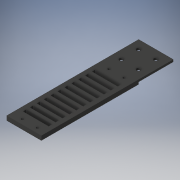
# Autodesk Inventor part: Base Right Front Panel
Saved by Autodesk Inventor 2019 (Build 230136000, 136)
## iProperties
Created: 2018-12-04
Part Number: Base Right Front Panel
Material: Generic
Document SubType Name: Modeling
Designer: Keith
Density: 1 g/cm^3
Appearance: Default
Author: Keith
## iProperties of the stored document Base Right Front Panel_3DPrint.ipt
Created: 2018-12-04
Part Number: Base Right Front Panel_3DPrint
Material: Generic
Document SubType Name: Modeling
Designer: Keith
Density: 1 g/cm^3
Appearance: Default
Author: Keith
Autodesk Inventor part; units mm, degrees
ref_plane "YZ Plane" through (0, 0, 0) normal (1, 0, 0) x (0, 1, 0)
ref_plane "XZ Plane" through (0, 0, 0) normal (0, 1, 0) x (-1, 0, 0)
ref_plane "XY Plane" through (0, 0, 0) normal (0, 0, 1) x (1, 0, 0)
sketch "Sketch1" plane through (0, 0, 0) normal (0, 1, 0) x (-1, 0, 0)
  line L0 (0, 0) -> (40, 0)
  line L1 (40, 0) -> (40, -152.8)
  line L2 (40, -152.8) -> (0, -152.8)
  line L3 (0, -152.8) -> (0, 0)
  circle A0 centre (30, -122.8) radius 2.5
  circle A1 centre (30, -142.8) radius 2.5
  circle A2 centre (10, -122.8) radius 2.5
  circle A3 centre (10, -142.8) radius 2.5
  line L4 (5, -97.55) -> (35, -97.55)
  line L5 (35, -97.55) -> (35, -93.55)
  line L6 (35, -93.55) -> (5, -93.55)
  line L7 (5, -93.55) -> (5, -97.55)
  line L8 (5, -89.55) -> (35, -89.55)
  line L9 (35, -89.55) -> (35, -85.55)
  line L10 (35, -85.55) -> (5, -85.55)
  line L11 (5, -85.55) -> (5, -89.55)
  line L12 (5, -81.55) -> (35, -81.55)
  line L13 (35, -81.55) -> (35, -77.55)
  line L14 (35, -77.55) -> (5, -77.55)
  line L15 (5, -77.55) -> (5, -81.55)
  line L16 (5, -73.55) -> (35, -73.55)
  line L17 (35, -73.55) -> (35, -69.55)
  line L18 (35, -69.55) -> (5, -69.55)
  line L19 (5, -69.55) -> (5, -73.55)
  line L20 (5, -65.55) -> (35, -65.55)
  line L21 (35, -65.55) -> (35, -61.55)
  line L22 (35, -61.55) -> (5, -61.55)
  line L23 (5, -61.55) -> (5, -65.55)
  line L24 (5, -57.55) -> (35, -57.55)
  line L25 (35, -57.55) -> (35, -53.55)
  line L26 (35, -53.55) -> (5, -53.55)
  line L27 (5, -53.55) -> (5, -57.55)
  line L28 (5, -49.55) -> (35, -49.55)
  line L29 (35, -49.55) -> (35, -45.55)
  line L30 (35, -45.55) -> (5, -45.55)
  line L31 (5, -45.55) -> (5, -49.55)
  line L32 (5, -41.55) -> (35, -41.55)
  line L33 (35, -41.55) -> (35, -37.55)
  line L34 (35, -37.55) -> (5, -37.55)
  line L35 (5, -37.55) -> (5, -41.55)
  line L36 (5, -33.55) -> (35, -33.55)
  line L37 (35, -33.55) -> (35, -29.55)
  line L38 (35, -29.55) -> (5, -29.55)
  line L39 (5, -29.55) -> (5, -33.55)
  line L40 (5, -25.55) -> (35, -25.55)
  line L41 (35, -25.55) -> (35, -21.55)
  line L42 (35, -21.55) -> (5, -21.55)
  line L43 (5, -21.55) -> (5, -25.55)
  line L44 (5, -17.55) -> (35, -17.55)
  line L45 (35, -17.55) -> (35, -13.55)
  line L46 (35, -13.55) -> (5, -13.55)
  line L47 (5, -13.55) -> (5, -17.55)
  dimension "d0" = 40
  dimension "d1" = 152.8
  dimension "d2" = 5
  dimension "d3" = 5
  dimension "d4" = 5
  dimension "d5" = 5
  dimension "d6" = 10
  dimension "d7" = 0
  dimension "d8" = 20
  dimension "d11" = 30
  dimension "d12" = 20
  dimension "d13" = 30
  dimension "d14" = 10
  dimension "d15" = 0
  dimension "d16" = 30
  dimension "d18" = 55.25
  dimension "d31" = 30
  dimension "d33" = 30
  dimension "d35" = 30
  dimension "d37" = 30
  dimension "d39" = 30
  dimension "d41" = 30
  dimension "d43" = 30
  dimension "d45" = 30
  dimension "d47" = 30
  dimension "d49" = 30
  constraints: 96 end point, 24 parallel, 12 horizontal, 12 perpendicular, 4 centre point
  measures "d0" distance of L1.end L2.end
  measures "d1" distance of L0.end L1.end
  measures "d2" diameter of A0
  measures "d3" diameter of A1
  measures "d4" diameter of A2
  measures "d5" diameter of A3
  measures "d6" distance from line of L1 A0.centre
  measures "d7" horizontal distance of A0.centre A1.centre
  measures "d8" distance of A0.centre A2.centre
  measures "d11" distance from line of L2 A0.centre
  measures "d12" distance of A1.centre A0.centre
  measures "d13" distance from line of L2 A2.centre
  measures "d14" distance from line of L2 A3.centre
  measures "d15" horizontal distance of A2.centre A3.centre
  measures "d16" distance of L6.end L5.end
  measures "d18" distance between parallel lines of L2 L4
  measures "d31" distance of L10.end L9.end
  measures "d33" distance of L14.end L13.end
  measures "d35" distance of L18.end L17.end
  measures "d37" distance of L22.end L21.end
  measures "d39" distance of L27.start L25.end
  measures "d41" distance of L31.start L29.end
  measures "d43" distance of L35.start L33.end
  measures "d45" distance of L39.start L37.end
  measures "d47" distance of L43.start L41.end
  measures "d49" distance of L47.start L45.end
extrude "Extrusion1" add sketch "Sketch1" along normal blind 5
sketch "Sketch2" plane through (0, 5, 0) normal (0, 1, 0) x (1, 0, 0)
  line L0 (-5, 17.55) -> (-5, 13.55) projected
  line L1 (-5, 13.55) -> (-35, 13.55) projected
  line L2 (-35, 13.55) -> (-35, 17.55) projected
  line L3 (-35, 17.55) -> (-5, 17.55) projected
  line L4 (-5, 25.55) -> (-5, 21.55) projected
  line L5 (-5, 21.55) -> (-35, 21.55) projected
  line L6 (-35, 21.55) -> (-35, 25.55) projected
  line L7 (-35, 25.55) -> (-5, 25.55) projected
  line L8 (-5, 33.55) -> (-5, 29.55) projected
  line L9 (-5, 29.55) -> (-35, 29.55) projected
  line L10 (-35, 29.55) -> (-35, 33.55) projected
  line L11 (-35, 33.55) -> (-5, 33.55) projected
  line L12 (-5, 41.55) -> (-5, 37.55) projected
  line L13 (-5, 37.55) -> (-35, 37.55) projected
  line L14 (-35, 37.55) -> (-35, 41.55) projected
  line L15 (-35, 41.55) -> (-5, 41.55) projected
  line L16 (-5, 49.55) -> (-5, 45.55) projected
  line L17 (-5, 45.55) -> (-35, 45.55) projected
  line L18 (-35, 45.55) -> (-35, 49.55) projected
  line L19 (-35, 49.55) -> (-5, 49.55) projected
  line L20 (-5, 57.55) -> (-5, 53.55) projected
  line L21 (-5, 53.55) -> (-35, 53.55) projected
  line L22 (-35, 53.55) -> (-35, 57.55) projected
  line L23 (-35, 57.55) -> (-5, 57.55) projected
  line L24 (-5, 65.55) -> (-5, 61.55) projected
  line L25 (-5, 61.55) -> (-35, 61.55) projected
  line L26 (-35, 61.55) -> (-35, 65.55) projected
  line L27 (-35, 65.55) -> (-5, 65.55) projected
  line L28 (-5, 73.55) -> (-5, 69.55) projected
  line L29 (-5, 69.55) -> (-35, 69.55) projected
  line L30 (-35, 69.55) -> (-35, 73.55) projected
  line L31 (-35, 73.55) -> (-5, 73.55) projected
  line L32 (-5, 81.55) -> (-5, 77.55) projected
  line L33 (-5, 77.55) -> (-35, 77.55) projected
  line L34 (-35, 77.55) -> (-35, 81.55) projected
  line L35 (-35, 81.55) -> (-5, 81.55) projected
  line L36 (-5, 89.55) -> (-5, 85.55) projected
  line L37 (-5, 85.55) -> (-35, 85.55) projected
  line L38 (-35, 85.55) -> (-35, 89.55) projected
  line L39 (-35, 89.55) -> (-5, 89.55) projected
  line L40 (-5, 97.55) -> (-5, 93.55) projected
  line L41 (-5, 93.55) -> (-35, 93.55) projected
  line L42 (-35, 93.55) -> (-35, 97.55) projected
  line L43 (-35, 97.55) -> (-5, 97.55) projected
  circle A0 centre (-10, 142.8) radius 2.5 projected
  circle A1 centre (-10, 122.8) radius 2.5 projected
  circle A2 centre (-30, 142.8) radius 2.5 projected
  circle A3 centre (-30, 122.8) radius 2.5 projected
  line L44 (-40, 0) -> (0, 0) projected
  line L45 (0, 0) -> (0, 152.8) projected
  line L46 (0, 152.8) -> (-40, 152.8) projected
  line L47 (-40, 152.8) -> (-40, 0) projected
  circle A4 centre (-27.5, 5.625) radius 1.5
  circle A5 centre (-10, 5.625) radius 1.5
  circle A6 centre (-27.5, 105.925) radius 1.5
  circle A7 centre (-10, 105.925) radius 1.5
  dimension "d53" = 3
  dimension "d54" = 3
  dimension "d55" = 3
  dimension "d56" = 3
  dimension "d57" = 12.5
  dimension "d58" = 10
  dimension "d59" = 12.5
  dimension "d60" = 10
  dimension "d61" = 5.625
  dimension "d62" = 5.625
  dimension "d63" = 46.875
  dimension "d64" = 46.875
  constraints: 4 centre point
  measures "d53" diameter of A4
  measures "d54" diameter of A5
  measures "d55" diameter of A6
  measures "d56" diameter of A7
  measures "d57" distance from line of L47 A4.centre
  measures "d58" distance from line of L45 A5.centre
  measures "d59" distance from line of L47 A6.centre
  measures "d60" distance from line of L45 A7.centre
  measures "d61" distance from line of L44 A4.centre
  measures "d62" distance from line of L44 A5.centre
  measures "d63" distance from line of L46 A6.centre
  measures "d64" distance from line of L46 A7.centre
extrude "Extrusion2" cut sketch "Sketch2" against normal blind 5 contours A4 | A5 | A6 | A7
sketch "Sketch3" plane through (0, 0, 0) normal (0, -1, 0) x (1, 0, 0)
  circle A0 centre (-27.5, -105.925) radius 1.5 projected
  circle A1 centre (-27.5, -5.625) radius 1.5 projected
  circle A2 centre (-10, -5.625) radius 1.5 projected
  circle A3 centre (-10, -105.925) radius 1.5 projected
  line L0 (-5, -13.55) -> (-5, -17.55) projected
  line L1 (-5, -17.55) -> (-35, -17.55) projected
  line L2 (-35, -17.55) -> (-35, -13.55) projected
  line L3 (-35, -13.55) -> (-5, -13.55) projected
  line L4 (-5, -21.55) -> (-5, -25.55) projected
  line L5 (-5, -25.55) -> (-35, -25.55) projected
  line L6 (-35, -25.55) -> (-35, -21.55) projected
  line L7 (-35, -21.55) -> (-5, -21.55) projected
  line L8 (-5, -29.55) -> (-5, -33.55) projected
  line L9 (-5, -33.55) -> (-35, -33.55) projected
  line L10 (-35, -33.55) -> (-35, -29.55) projected
  line L11 (-35, -29.55) -> (-5, -29.55) projected
  line L12 (-5, -37.55) -> (-5, -41.55) projected
  line L13 (-5, -41.55) -> (-35, -41.55) projected
  line L14 (-35, -41.55) -> (-35, -37.55) projected
  line L15 (-35, -37.55) -> (-5, -37.55) projected
  line L16 (-5, -45.55) -> (-5, -49.55) projected
  line L17 (-5, -49.55) -> (-35, -49.55) projected
  line L18 (-35, -49.55) -> (-35, -45.55) projected
  line L19 (-35, -45.55) -> (-5, -45.55) projected
  line L20 (-5, -53.55) -> (-5, -57.55) projected
  line L21 (-5, -57.55) -> (-35, -57.55) projected
  line L22 (-35, -57.55) -> (-35, -53.55) projected
  line L23 (-35, -53.55) -> (-5, -53.55) projected
  line L24 (-5, -61.55) -> (-5, -65.55) projected
  line L25 (-5, -65.55) -> (-35, -65.55) projected
  line L26 (-35, -65.55) -> (-35, -61.55) projected
  line L27 (-35, -61.55) -> (-5, -61.55) projected
  line L28 (-5, -69.55) -> (-5, -73.55) projected
  line L29 (-5, -73.55) -> (-35, -73.55) projected
  line L30 (-35, -73.55) -> (-35, -69.55) projected
  line L31 (-35, -69.55) -> (-5, -69.55) projected
  line L32 (-5, -77.55) -> (-5, -81.55) projected
  line L33 (-5, -81.55) -> (-35, -81.55) projected
  line L34 (-35, -81.55) -> (-35, -77.55) projected
  line L35 (-35, -77.55) -> (-5, -77.55) projected
  line L36 (-5, -85.55) -> (-5, -89.55) projected
  line L37 (-5, -89.55) -> (-35, -89.55) projected
  line L38 (-35, -89.55) -> (-35, -85.55) projected
  line L39 (-35, -85.55) -> (-5, -85.55) projected
  line L40 (-5, -93.55) -> (-5, -97.55) projected
  line L41 (-5, -97.55) -> (-35, -97.55) projected
  line L42 (-35, -97.55) -> (-35, -93.55) projected
  line L43 (-35, -93.55) -> (-5, -93.55) projected
  circle A4 centre (-10, -142.8) radius 2.5 projected
  circle A5 centre (-10, -122.8) radius 2.5 projected
  circle A6 centre (-30, -142.8) radius 2.5 projected
  circle A7 centre (-30, -122.8) radius 2.5 projected
  line L44 (0, 0) -> (-40, 0) projected
  line L45 (-40, 0) -> (-40, -152.8) projected
  line L46 (-40, -152.8) -> (0, -152.8) projected
  line L47 (0, -152.8) -> (0, 0) projected
  line L48 (0, 0) -> (0, -152.8) projected
  line L49 (-40, -152.8) -> (0, -152.8)
  line L50 (0, -152.8) -> (0, -112.8)
  line L51 (0, -112.8) -> (-40, -112.8)
  line L52 (-40, -112.8) -> (-40, -152.8)
  dimension "d67" = 40
  constraints: 8 end point, 2 parallel, 1 horizontal, 1 perpendicular, 1 point on line
  measures "d67" distance of L50.end L49.end
extrude "Extrusion3" cut sketch "Sketch3" against normal blind 2.5 contours L47 L46 L45 L51
body "Solid1"
